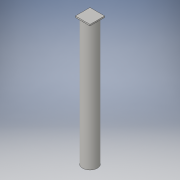
# Autodesk Inventor part: bottom hook
Saved by Autodesk Inventor 2016 (Build 200138000, 138)
## iProperties
Created: 2016-01-16
Part Number: bottom hook
Material: Generic
Document SubType Name: Modeling
Designer: Administrator
Density: 1 g/cm^3
Appearance: Default
Author: Administrator
Autodesk Inventor part; units mm, degrees
ref_plane "YZ Plane" through (0, 0, 0) normal (1, 0, 0) x (0, 1, 0)
ref_plane "XZ Plane" through (0, 0, 0) normal (0, 1, 0) x (-1, 0, 0)
ref_plane "XY Plane" through (0, 0, 0) normal (0, 0, 1) x (1, 0, 0)
sketch "Sketch1" plane through (0, 0, 0) normal (0, 1, 0) x (-1, 0, 0)
  circle A0 centre (0, 0) radius 2.9337
  dimension "d0" = 5.8674
  constraints: 1 centre point, 1 coincident
  measures "d0" diameter of A0
extrude "Extrusion1" add sketch "Sketch1" along normal blind 50.8
sketch "Sketch2" plane through (0, 50.8, 0) normal (0, 1, 0) x (1, 0, 0)
  line L0 (-2.9337, 2.9337) -> (2.9337, 2.9337)
  line L1 (2.9337, 2.9337) -> (2.9337, -2.9337)
  line L2 (2.9337, -2.9337) -> (-2.9337, -2.9337)
  line L3 (-2.9337, -2.9337) -> (-2.9337, 2.9337)
  line L4 (-2.9337, 2.9337) -> (2.9337, -2.9337) construction
  line L5 (2.9337, 2.9337) -> (-2.9337, -2.9337) construction
  point P0 (0, 0)
  dimension "d3" = 5.8674
  dimension "d4" = 5.8674
  constraints: 12 end point, 2 midpoint, 2 parallel, 1 horizontal, 1 perpendicular
  measures "d3" distance of L1.end L2.end
  measures "d4" distance of L0.end L1.end
extrude "Extrusion2" add sketch "Sketch2" along normal blind 0.508
body "Solid1"
